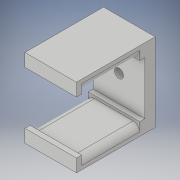
# Autodesk Inventor part: chain tensioner
Saved by Autodesk Inventor 2019 (Build 230136000, 136)
## iProperties
Created: 2019-09-24
Part Number: chain tensioner
Material: Generic
Document SubType Name: Modeling
Designer: Delta
Density: 1 g/cm^3
Appearance: Default
Author: Delta
Autodesk Inventor part; units mm, degrees
ref_plane "YZ Plane" through (0, 0, 0) normal (1, 0, 0) x (0, 1, 0)
ref_plane "XZ Plane" through (0, 0, 0) normal (0, 1, 0) x (-1, 0, 0)
ref_plane "XY Plane" through (0, 0, 0) normal (0, 0, 1) x (1, 0, 0)
sketch "Sketch1" plane through (0, 0, 0) normal (0, 0, 1) x (1, 0, 0)
  line L0 (0, 0) -> (-25.4, 0)
  line L1 (-25.4, 0) -> (-25.4, 38.735)
  line L2 (-25.4, 38.735) -> (0, 38.735)
  line L3 (0, 38.735) -> (0, 0)
  dimension "d0" = 25.4
  dimension "d1" = 38.735
  constraints: 8 end point, 2 parallel, 1 horizontal, 1 perpendicular
  measures "d0" distance between parallel lines of L3 L1
  measures "d1" distance of L2.end L0.start
extrude "Extrusion1" add sketch "Sketch1" along normal blind 7.62
sketch "Sketch5" plane through (0, 0, 7.62) normal (0, 0, 1) x (1, 0, 0)
  line L0 (-25.4, 0) -> (0, 0) projected
  line L1 (-25.4, 38.735) -> (-25.4, 0) projected
  line L2 (0, 0) -> (-25.4, 0)
  line L3 (-25.4, 0) -> (-25.4, 5.08)
  line L4 (-25.4, 5.08) -> (0, 5.08)
  line L5 (0, 5.08) -> (0, 0)
  line L6 (0, 38.735) -> (-25.4, 38.735)
  line L7 (-25.4, 38.735) -> (-25.4, 33.655)
  line L8 (-25.4, 33.655) -> (0, 33.655)
  line L9 (0, 33.655) -> (0, 38.735)
  line L10 (0, 38.735) -> (-25.4, 38.735) projected
  dimension "d29" = 5.08
  dimension "d30" = 5.08
  dimension "d31" = 0
  constraints: 16 end point, 4 parallel, 3 point on line, 2 horizontal, 2 perpendicular
  measures "d29" distance of L2.end L3.end
  measures "d30" distance between parallel lines of L6 L8
  measures "d31" distance between parallel lines of L10 L6
extrude "Extrusion4" add sketch "Sketch5" along normal blind 28.575
sketch "Sketch6" plane through (0, 0, 36.195) normal (0, 0, 1) x (1, 0, 0)
  line L0 (-25.4, 0) -> (-25.4, 38.735) projected
  line L1 (-25.4, 38.735) -> (0, 38.735)
  line L2 (0, 38.735) -> (0, 32.385)
  line L3 (0, 32.385) -> (-25.4, 32.385)
  line L4 (-25.4, 32.385) -> (-25.4, 38.735)
  line L5 (-25.4, 0) -> (0, 0)
  line L6 (0, 0) -> (0, 6.35)
  line L7 (0, 6.35) -> (-25.4, 6.35)
  line L8 (-25.4, 6.35) -> (-25.4, 0)
  line L9 (-25.4, 33.655) -> (0, 33.655) projected
  dimension "d34" = 5.08
  dimension "d35" = 6.35
  dimension "d36" = 6.35
  dimension "d37" = 25.4
  dimension "d38" = 25.4
  constraints: 16 end point, 4 parallel, 2 horizontal, 2 perpendicular
  measures "d34" distance between parallel lines of L1 L9
  measures "d35" distance between parallel lines of L3 L1
  measures "d36" distance between parallel lines of L5 L7
  measures "d37" distance between parallel lines of L0 L6
  measures "d38" distance between parallel lines of L0 L2
extrude "Extrusion5" add sketch "Sketch6" along normal blind 2.54
sketch "Sketch7" plane through (0, 0, 7.62) normal (0, 0, 1) x (1, 0, 0)
  line L0 (-25.4, 33.655) -> (-25.4, 5.08) projected
  line L1 (-25.4, 32.385) -> (0, 32.385)
  line L2 (0, 32.385) -> (0, 6.35)
  line L3 (0, 6.35) -> (-25.4, 6.35)
  line L4 (-25.4, 6.35) -> (-25.4, 32.385)
  line L5 (-25.4, 5.08) -> (0, 5.08) projected
  point P0 (0, 0)
  dimension "d41" = 26.035
  dimension "d42" = 1.27
  dimension "d43" = 25.4
  constraints: 8 end point, 2 parallel, 1 horizontal, 1 perpendicular, 1 point on line
  measures "d41" distance between parallel lines of L3 L1
  measures "d42" distance between parallel lines of L5 L3
  measures "d43" distance between parallel lines of L2 L0
extrude "Extrusion6" cut sketch "Sketch7" against normal blind 2.54
fillet "Fillet2" radius 3.175 4 edges at (0, 33.655, 21.9075) (-25.4, 33.655, 21.9075) (-25.4, 5.08, 21.9075) (0, 5.08, 21.9075)
sketch "Sketch8" plane through (0, 0, 0) normal (0, 0, -1) x (-1, 0, 0)
  line L0 (25.4, 0) -> (25.4, 38.735) projected
  line L1 (0, 38.735) -> (0, 0) projected
  line L2 (25.4, 38.735) -> (0, 38.735) projected
  line L3 (0, 0) -> (25.4, 0) projected
  point P0 (12.7, 19.3675)
  dimension "d47" = 12.7
  dimension "d48" = 25.4
  dimension "d49" = 38.735
  dimension "d50" = 19.3675
  measures "d47" distance from line of L0 point (12.7, 19.367)
  measures "d48" distance between parallel lines of L0 L1
  measures "d49" distance between parallel lines of L2 L3
  measures "d50" distance from line of L2 point (12.7, 19.367)
hole "Hole2" at (-12.7, 19.3675, 0) direction (0, 0, 1) diameter 4.4958 end through all clearance for "Flat Head Machine Screw (82)" size "#8" standard "Ansi Unified Screw Threads"
equation "\"d30\" = d29"
equation "\"d36\" = d35"
equation "\"d47\" = 0.5 * d48"
equation "\"d50\" = 0.5 * d49"
body "Solid1"
